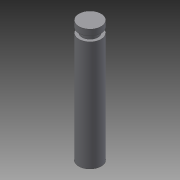
# Autodesk Inventor part: Fixture_Weight_Shaft
Saved by Autodesk Inventor 2015 (Build 190159000, 159)
## iProperties
Created: 2015-01-18
Part Number: Fixture_Weight_Shaft
Material: Generic
Document SubType Name: Modeling
Designer: Drew
Density: 1 g/cm^3
Appearance: Default
Author: Drew
Autodesk Inventor part; units mm, degrees
ref_plane "YZ Plane" through (0, 0, 0) normal (1, 0, 0) x (0, 1, 0)
ref_plane "XZ Plane" through (0, 0, 0) normal (0, 1, 0) x (-1, 0, 0)
ref_plane "XY Plane" through (0, 0, 0) normal (0, 0, 1) x (1, 0, 0)
sketch "Sketch1" plane through (0, 0, 0) normal (0, 0, 1) x (1, 0, 0)
  line L0 (0, 0) -> (0, 34.5188)
  line L1 (0, 34.5188) -> (3.175, 34.5188)
  line L2 (3.175, 34.5188) -> (3.175, 32.8429)
  line L3 (3.175, 32.8429) -> (2.2578, 32.8429)
  line L4 (2.2578, 32.8429) -> (2.2578, 31.3755)
  line L5 (2.2578, 31.3755) -> (3.175, 31.3755)
  line L6 (3.175, 31.3755) -> (3.175, 0)
  line L7 (3.175, 0) -> (0, 0)
  dimension "d0" = 3.175
  dimension "d1" = 34.5188
  dimension "d2" = 1.4674
  dimension "d3" = 0.9172
  dimension "d4" = 1.6759
  constraints: 16 end point, 6 perpendicular, 2 point on line, 1 vertical
  measures "d0" distance of L0.end L1.end
  measures "d1" distance between parallel lines of L7 L1
  measures "d2" distance between parallel lines of L5 L3
  measures "d3" distance between parallel lines of L4 L2
  measures "d4" distance between parallel lines of L1 L3
revolve "Revolution1" add sketch "Sketch1" angle 360 about axis through (0, 0, 0) along (0, 1, 0)
body "Solid1"
